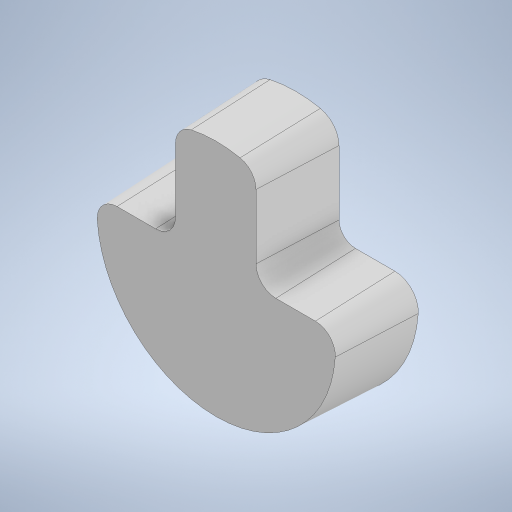
# Autodesk Inventor part: Crank Cast Image
Saved by Autodesk Inventor 2023 (Build 270158000, 158)
## iProperties
Created: 2022-12-28
Part Number: Crank Cast Image
Material: Generic
Document SubType Name: Modeling
Designer: tgr41
Density: 1 g/cm^3
Appearance: Default
Author: tgr41
Autodesk Inventor part; units mm, degrees
ref_plane "YZ Plane" through (0, 0, 0) normal (1, 0, 0) x (0, 1, 0)
ref_plane "XZ Plane" through (0, 0, 0) normal (0, 1, 0) x (-1, 0, 0)
ref_plane "XY Plane" through (0, 0, 0) normal (0, 0, 1) x (1, 0, 0)
sketch "Sketch1" plane through (0, 0, 0) normal (0, 0, 1) x (1, 0, 0)
  circle A0 centre (0, 12.7) radius 3.175
  circle A1 centre (-0.0751, 0) radius 3.175
  line L0 (-0.0751, 0) -> (-0.0751, 19.0499)
  line L1 (-0.0751, 3.175) -> (-0.0751, 24.8386)
  line L2 (6.35, 15.5543) -> (6.35, 5.2605)
  line L3 (9.525, 2.0855) -> (15.8376, 2.0855)
  line L4 (-6.5001, 15.5229) -> (-6.5001, 5.2772)
  line L5 (-9.6751, 2.1022) -> (-15.8387, 2.1022)
  arc A2 (-19.0064, -1.2874) -> (19.0051, -1.3074) centre (0, 0) ccw
  arc A3 (3.81, 18.6651) -> (-3.9901, 18.6274) centre (0, 0) ccw
  arc A4 (-3.9901, 18.6274) -> (-6.5001, 15.5229) centre (-3.3251, 15.5229) ccw
  arc A5 (6.35, 15.5543) -> (3.81, 18.6651) centre (3.175, 15.5543) ccw
  arc A6 (6.35, 5.2605) -> (9.525, 2.0855) centre (9.525, 5.2605) ccw
  arc A7 (-9.6751, 2.1022) -> (-6.5001, 5.2772) centre (-9.6751, 5.2772) ccw
  arc A8 (-15.8387, 2.1022) -> (-19.0064, -1.2874) centre (-15.8387, -1.0728) ccw
  arc A9 (19.0051, -1.3074) -> (15.8376, 2.0855) centre (15.8376, -1.0895) ccw
  point P0 (6.35, 17.9605)
  point P1 (6.35, 2.0855)
  point P2 (18.9355, 2.0855)
  point P3 (-6.5001, 2.1022)
  point P4 (-18.9337, 2.1022)
  point P5 (-6.5001, 17.9067)
  dimension "d6" = 6.35
  dimension "d3" = 6.35
  dimension "d11" = 15.875
  dimension "d12" = 3.175
  constraints: 21 point on circle, 12 end point, 12 tangent, 10 point on line, 9 centre point, 5 equal radius, 2 perpendicular, 1 coincident, 1 vertical, 1 vertical alignment, 2 other
  measures "d3" diameter of A0
  measures "d11" distance of point (6.35, 17.961) point (6.35, 2.086)
  measures "d12" radius of A4
extrude "Extrusion1" add sketch "Sketch1" along normal blind 12.7 contours A0 L0 | L0 A0 | A1 | L2 A6 L3 A9 A2 A8 L5 A7 L4 A4 A3 A5
draft "FaceDraft1" angle 2.5 pull direction (0, 0, 1) faces at (6.35, 8.6918, 4.2333) (4.713, 18.3319, 8.4667) (6.5695, 4.1006, 8.4667) (2.9511, 18.82, 4.2333) (13.7334, 2.0855, 4.2333) (-6.0664, 17.1247, 8.4667) (16.3313, 2.0469, 8.4667) (-6.5001, 12.1076, 4.2333) (18.5791, -4.2093, 8.4667) (-7.8866, 2.6539, 8.4667) (-16.0862, 2.0925, 4.2333) (-11.7296, 2.1022, 4.2333) fixed edges at (6.35, 10.4074, 12.7) (5.6343, 17.5623, 12.7) (7.2799, 3.0154, 12.7) (-0.092, 19.0498, 12.7) (12.6813, 2.0855, 12.7) (-5.7941, 17.519, 12.7) (18.1584, 1.0772, 12.7) (-6.5001, 10.4, 12.7) (-0.01, -19.05, 12.7) (-7.43, 3.0321, 12.7) (-18.1584, 1.0951, 12.7) (-12.7569, 2.1022, 12.7)
body "Solid1"
